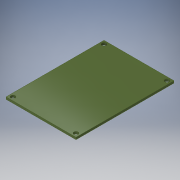
# Autodesk Inventor part: КВ33.044.1002 - Плата распределительная
Saved by Autodesk Inventor 2019 (Build 230136000, 136)
## iProperties
Created: 2019-10-30
Part Number: КВ33.044.1002 - Плата распределительная
Material: Серебро
Document SubType Name: Modeling
Designer: Петров Иван
Density: 10.49 g/cm^3
Appearance: Темно-оливковый
Author: Петров Иван
Autodesk Inventor part; units mm, degrees
ref_plane "YZ Plane" through (0, 0, 0) normal (1, 0, 0) x (0, 1, 0)
ref_plane "XZ Plane" through (0, 0, 0) normal (0, 1, 0) x (-1, 0, 0)
ref_plane "XY Plane" through (0, 0, 0) normal (0, 0, 1) x (1, 0, 0)
sketch "Эскиз1" plane through (0, 0, 0) normal (0, 1, 0) x (-1, 0, 0)
  line L0 (-25, 35) -> (25, 35)
  line L1 (25, 35) -> (25, -35)
  line L2 (25, -35) -> (-25, -35)
  line L3 (-25, -35) -> (-25, 35)
  circle A0 centre (22.5, 32.5) radius 1.5
  circle A1 centre (22.5, -32.5) radius 1.5
  circle A2 centre (-22.5, -32.5) radius 1.5
  circle A3 centre (-22.5, 32.5) radius 1.5
  point P0 (0, 0)
  dimension "d0" = 50
  dimension "d1" = 70
  dimension "d4" = 3
  dimension "d5" = 3
  dimension "d6" = 3
  dimension "d7" = 3
  constraints: 8 end point, 4 centre point, 2 parallel, 1 horizontal, 1 perpendicular
  measures "d0" distance of L1.end L2.end
  measures "d1" distance of L0.end L1.end
  measures "d4" diameter of A0
  measures "d5" diameter of A1
  measures "d6" diameter of A2
  measures "d7" diameter of A3
extrude "Выдавливание1" add sketch "Эскиз1" along normal blind 1.5
